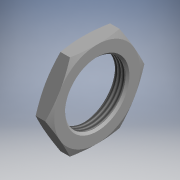
# Autodesk Inventor part: Nut M18 x 1
Saved by Autodesk Inventor 2017.3 (Build 213256000, 256)
## iProperties
Part Number: Nut M18 x 1
Material: Generic
Catalog Web Link: www.cadenas.de
Description: Nut M18 x 1-Balluf - Inductive Sensor
Vendor: BALLUFF
Document SubType Name: Modeling
Designer: partserver
Manufacturer: BALLUFF
Mass: 1.06141 g
Surface Area: 10.2773 cm^2
Volume: 1.06141 cm^3
Density: 1 g/cm^3
Appearance: PSOLRGB-192-192-192
Category: PARTsolutions
Company: BALLUFF
Title: Nut M18 x 1
Author: Cadenas PARTsolutions
Comments: Balluf - Inductive Sensor
PSOL_IDENT_0: {$CADENAS_DATA\23d-libs\balluff\sensortechnik\induktiv\dc_3_4_draht\mutter_m18x1.prj},169 {VTYP=3D},
PSOL_IDENT_1: {NB=Nut M18 x 1},{LINA=Nut M18 x 1},{NN=Nut M18 x 1},{DATE=15.02.2021 12:07:22},{GEOMDATE=03.05.2019
PSOL_IDENT_2: 06:10:00},{VERSION=v1},{LINEID=10},{WBVAR=},{WBNUMERIC=}  {NB=MUTTER M18 x 1},{LINA=MUTTER M18 x 1}
PSOL_IDENT_3: ,{KT=DUMMY},{AB=MUTTER M18 x 1},{AB1=MUTTER_M18_x_1},{VISONPSERV=0.000}
NB: Nut M18 x 1
NN: Nut M18 x 1
NT: Balluf - Inductive Sensor
NBSYN: Nut M18 x 1
LINA: Nut M18 x 1
CATALOG: Balluff
AB: MUTTER M18 x 1
VISONPSERV: 0
SUPPLIER: BALLUFF
ARTICLENO: Nut M18 x 1
BOMINFO: Nut M18 x 1
CREATOR: CADENAS GmbH
Autodesk Inventor part; units mm, degrees
sketch "Skizze_1" plane through (0, 0, 0) normal (0, 0, 1) x (1, 0, 0)
  line L0 (2, 0) -> (-2, 0)
  line L1 (-2, 0) -> (-2, 12)
  line L2 (-2, 12) -> (-1.1265, 14.4)
  line L3 (-1.1265, 14.4) -> (1.1265, 14.4)
  line L4 (1.1265, 14.4) -> (2, 12)
  line L5 (2, 12) -> (2, 0)
  line L6 (2, 0) -> (-2, 0)
  constraints: 14 end point
revolve "Revolution1" add sketch "Skizze_1" angle 360 about axis through (2, 0, 0) along (-1, 0, 0)
sketch "Skizze_2" plane through (0, 0, 0) normal (1, 0, 0) x (0, 1, 0)
  line L0 (24, 24) -> (-24, 24)
  line L1 (-24, 24) -> (-24, -24)
  line L2 (-24, -24) -> (24, -24)
  line L3 (24, -24) -> (24, 24)
  line L4 (-6.9282, 12) -> (-13.8564, 0)
  line L5 (-13.8564, 0) -> (-6.9282, -12)
  line L6 (-6.9282, -12) -> (6.9282, -12)
  line L7 (6.9282, -12) -> (13.8564, 0)
  line L8 (13.8564, 0) -> (6.9282, 12)
  line L9 (6.9282, 12) -> (-6.9282, 12)
  constraints: 20 end point
extrude "Extrusion1" cut sketch "Skizze_2" along normal mid plane 8
sketch "Skizze_3" plane through (0, 0, 0) normal (0, 0, 1) x (1, 0, 0)
  line L0 (2, 0) -> (-2, 0)
  line L1 (-2, 0) -> (-2, 9)
  line L2 (-2, 9) -> (-1.4585, 8.4585)
  line L3 (-1.4585, 8.4585) -> (1.4585, 8.4585)
  line L4 (1.4585, 8.4585) -> (2, 9)
  line L5 (2, 9) -> (2, 0)
  line L6 (2, 0) -> (-2, 0)
  constraints: 14 end point
revolve "Revolution2" cut sketch "Skizze_3" angle 360 about axis through (2, 0, 0) along (-1, 0, 0)
thread "Thread1" size "M18x1" class "6H" standard "ISO Metric profile" full length
ref_plane "m18_XY" through (0, 0, 0) normal (1, 0, 0) x (0, 0, -1)
ref_plane "m18_YZ" through (0, 0, 0) normal (0, 0, -1) x (0, 1, 0)
ref_plane "m18_ZX" through (0, 0, 0) normal (0, 1, 0) x (1, 0, 0)
body "Solid1"
